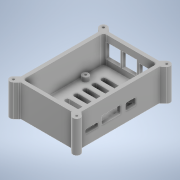
# Autodesk Inventor part: Case RevB Short
Saved by Autodesk Inventor 2021 (Build 250183000, 183)
## iProperties
Created: 2021-07-24
Part Number: Case RevB Short
Material: ABS Plastic
Document SubType Name: Modeling
Designer: cmzgt
Density: 0.1 g/cm^3
Appearance: Smooth - White
Author: cmzgt
## iProperties of the stored document _3DPrint.ipt
Created: 2021-07-24
Part Number: _3DPrint
Material: Generic
Document SubType Name: Modeling
Designer: cmzgt
Density: 1 g/cm^3
Appearance: Default
Author: cmzgt
Autodesk Inventor part; units mm, degrees
ref_plane "YZ Plane" through (0, 0, 0) normal (1, 0, 0) x (0, 1, 0)
ref_plane "XZ Plane" through (0, 0, 0) normal (0, 1, 0) x (-1, 0, 0)
ref_plane "XY Plane" through (0, 0, 0) normal (0, 0, 1) x (1, 0, 0)
sketch "Sketch1" plane through (0, 0, 0) normal (0, 1, 0) x (-1, 0, 0)
  line L0 (-33.3, -48.25) -> (33.3, -48.25)
  line L1 (33.3, -48.25) -> (33.3, 48.25)
  line L2 (33.3, 48.25) -> (-33.3, 48.25)
  line L3 (-33.3, 48.25) -> (-33.3, -48.25)
  line L4 (-33.3, -48.25) -> (33.3, 48.25) construction
  line L5 (33.3, -48.25) -> (-33.3, 48.25) construction
  point P0 (0, 0)
  dimension "d0" = 66.6
  dimension "d1" = 96.5
  constraints: 12 end point, 2 midpoint, 2 parallel, 1 horizontal, 1 perpendicular
  measures "d0" distance of L2.end L1.end
  measures "d1" distance of L0.end L1.end
extrude "Extrusion1" add sketch "Sketch1" along normal blind 5.08
sketch "Sketch2" plane through (0, 5.08, 0) normal (0, 1, 0) x (1, 0, 0)
  line L0 (29.5, 44.45) -> (-29.5, 44.45)
  line L1 (-29.5, 44.45) -> (-29.5, -44.45)
  line L2 (-29.5, -44.45) -> (29.5, -44.45)
  line L3 (29.5, -44.45) -> (29.5, 44.45)
  line L4 (29.5, 44.45) -> (-29.5, -44.45) construction
  line L5 (-29.5, 44.45) -> (29.5, -44.45) construction
  line L6 (-33.3, 48.25) -> (-33.3, -48.25) projected
  line L7 (-33.3, -48.25) -> (33.3, -48.25) projected
  line L8 (33.3, 48.25) -> (-33.3, 48.25) projected
  line L9 (33.3, -48.25) -> (33.3, 48.25) projected
  line L10 (25.7, -40.65) -> (33.3, -48.25) construction
  line L11 (23.8431, -44.45) -> (30.4716, -51.0784)
  line L12 (36.1284, -45.4216) -> (29.5, -38.7931)
  arc A0 (30.4716, -51.0784) -> (36.1284, -45.4216) centre (33.3, -48.25) ccw
  circle A1 centre (33.3, -48.25) radius 1.375
  point P0 (0, 0)
  dimension "d4" = 3.8
  dimension "d5" = 3.8
  dimension "d22" = 8
  dimension "d23" = 2.75
  constraints: 20 end point, 4 parallel, 3 midpoint, 2 centre point, 2 point on circle, 2 point on line, 2 tangent, 1 coincident, 1 horizontal, 1 perpendicular
  measures "d4" distance between parallel lines of L6 L1
  measures "d5" distance between parallel lines of L7 L2
  measures "d22" diameter of A0
  measures "d23" diameter of A1
extrude "Extrusion2" add sketch "Sketch2" along normal blind 30 contours L0 L1 L2 L11 L7 L6 L8 L9 L12 L3 | L12 L9 A1 L7 L11 L2 L3 | L9 L7 A1 picked at (32.8154, -47.4787)
sketch "Sketch3" plane through (0, 5.08, 0) normal (0, 1, 0) x (1, 0, 0)
  line L0 (29.5, -44.45) -> (-29.5, -44.45) construction
  line L1 (0, -44.45) -> (0, 44.45) construction
  line L2 (29.5, 44.45) -> (-29.5, 44.45) construction
  circle A0 centre (-24.5, -38.45) radius 3.5
  circle A1 centre (-24.5, -38.45) radius 1.375
  line L3 (29.5, 44.45) -> (29.5, -44.45) construction
  line L4 (29.5, 0) -> (-29.5, 0) construction
  line L5 (-29.5, -44.45) -> (-29.5, 44.45) construction
  circle A2 centre (-24.5, 19.55) radius 3.5
  circle A3 centre (-24.5, 19.55) radius 1.375
  circle A4 centre (24.5, -38.45) radius 3.5
  circle A5 centre (24.5, -38.45) radius 1.375
  circle A6 centre (24.5, 19.55) radius 3.5
  circle A7 centre (24.5, 19.55) radius 1.375
  point P0 (0, 0)
  dimension "d8" = 7
  dimension "d9" = 2.75
  dimension "d10" = 6
  dimension "d11" = 24.5
  dimension "d14" = 58
  constraints: 8 centre point, 4 coincident, 4 end point, 4 midpoint, 4 symmetric about line, 1 vertical, 8 other
  measures "d8" diameter of A0
  measures "d9" diameter of A1
  measures "d10" distance from line of L0 A0.centre
  measures "d11" distance from line of L1 A1.centre
  measures "d14" distance of A0.centre A2.centre
extrude "Extrusion3" add sketch "Sketch3" along normal blind 5
sketch "Sketch4" plane through (0, 0, 0) normal (0, -1, 0) x (1, 0, 0)
  line L0 (31.7938, 46.9342) -> (34.8062, 49.5658) construction
  line L1 (33.3, 48.25) -> (33.3, -48.25) projected
  line L2 (33.3, 42.9386) -> (37.4378, 46.5534)
  line L3 (32.1745, 52.5782) -> (29.1622, 49.9466)
  arc A0 (29.1622, 49.9466) -> (28.0164, 48.25) centre (31.7938, 46.9342) ccw
  arc A1 (37.4378, 46.5534) -> (32.1745, 52.5782) centre (34.8062, 49.5658) ccw
  line L4 (-33.3, 48.25) -> (33.3, 48.25) projected
  line L5 (28.0164, 48.25) -> (33.3, 48.25)
  line L6 (33.3, 48.25) -> (33.3, 42.9386)
  circle A2 centre (34.8062, 49.5658) radius 1.375
  line L7 (0, 48.25) -> (0, -48.25) construction
  line L8 (33.3, -48.25) -> (-33.3, -48.25) construction
  line L9 (33.3, 0) -> (-33.3, 0) construction
  line L10 (33.3, -48.25) -> (33.3, 48.25)
  line L11 (33.3, -42.9386) -> (37.4378, -46.5534)
  line L12 (32.1745, -52.5782) -> (29.1622, -49.9466)
  arc A3 (28.0164, -48.25) -> (29.1622, -49.9466) centre (31.7938, -46.9342) ccw
  arc A4 (32.1745, -52.5782) -> (37.4378, -46.5534) centre (34.8062, -49.5658) ccw
  line L13 (-33.3, -48.25) -> (33.3, -48.25)
  circle A5 centre (34.8062, -49.5658) radius 1.375
  line L14 (-33.3, 48.25) -> (-33.3, -48.25)
  line L15 (-33.3, 42.9386) -> (-37.4378, 46.5534)
  line L16 (-32.1745, 52.5782) -> (-29.1622, 49.9466)
  arc A6 (-28.0164, 48.25) -> (-29.1622, 49.9466) centre (-31.7938, 46.9342) ccw
  arc A7 (-32.1745, 52.5782) -> (-37.4378, 46.5534) centre (-34.8062, 49.5658) ccw
  line L17 (-28.0164, 48.25) -> (-33.3, 48.25)
  circle A8 centre (-34.8062, 49.5658) radius 1.375
  arc A9 (-37.4378, -46.5534) -> (-32.1745, -52.5782) centre (-34.8062, -49.5658) ccw
  line L18 (-33.3, -42.9386) -> (-37.4378, -46.5534)
  line L19 (-32.1745, -52.5782) -> (-29.1622, -49.9466)
  arc A10 (-29.1622, -49.9466) -> (-28.0164, -48.25) centre (-31.7938, -46.9342) ccw
  circle A11 centre (-34.8062, -49.5658) radius 1.375
  line L20 (-28.0164, -48.25) -> (-33.3, -48.25)
  line L21 (-33.3, -48.25) -> (-33.3, 48.25)
  point P0 (0, 0)
  point P1 (-28.0164, -48.25)
  point P2 (-33.3, -42.9386)
  point P3 (-28.0164, 48.25)
  point P4 (33.3, -42.9386)
  dimension "d24" = 2
  dimension "d25" = 8
  dimension "d26" = 131.141
  dimension "d27" = 2.75
  constraints: 40 end point, 30 symmetric about line, 16 point on circle, 12 centre point, 6 point on line, 4 coincident, 4 midpoint, 4 tangent, 1 collinear, 1 horizontal, 1 parallel, 9 other
  measures "d24" distance of L1.start L0.end
  measures "d25" diameter of A1
  measures "d26" angle of L1 L2
  measures "d27" diameter of A2
extrude "Extrusion4" add sketch "Sketch4" against normal up to surface (35.08 mm away) contours L4 A0 L3 A1 L2 L1 | L11 A4 L12 A3 L13 L1 | L4 L14 L15 A7 L16 A6 | A10 L19 A9 L18 L14 L13
fillet "Fillet2" radius 3 4 edges at (29.5, 20.08, -44.45) (-29.5, 20.08, -44.45) (-29.5, 20.08, 44.45) (29.5, 20.08, 44.45)
sketch "Sketch5" plane through (0, 5.08, 0) normal (0, 1, 0) x (1, 0, 0)
  line L0 (15, 0) -> (-15, 0) construction
  line L1 (15, 2.5) -> (-15, 2.5)
  line L2 (-15, -2.5) -> (15, -2.5)
  arc A0 (15, -2.5) -> (15, 2.5) centre (15, 0) ccw
  arc A1 (-15, 2.5) -> (-15, -2.5) centre (-15, 0) ccw
  line L3 (-26.5, -44.45) -> (26.5, -44.45) construction
  line L4 (0, -44.45) -> (0, 44.45) construction
  line L5 (-26.5, 44.45) -> (26.5, 44.45) construction
  arc A2 (-15, 12.5) -> (-15, 7.5) centre (-15, 10) ccw
  line L6 (15, 12.5) -> (-15, 12.5)
  line L7 (-15, 7.5) -> (15, 7.5)
  arc A3 (15, 7.5) -> (15, 12.5) centre (15, 10) ccw
  arc A4 (-15, 22.5) -> (-15, 17.5) centre (-15, 20) ccw
  line L8 (15, 22.5) -> (-15, 22.5)
  line L9 (-15, 17.5) -> (15, 17.5)
  arc A5 (15, 17.5) -> (15, 22.5) centre (15, 20) ccw
  arc A6 (-15, 32.5) -> (-15, 27.5) centre (-15, 30) ccw
  line L10 (15, 32.5) -> (-15, 32.5)
  line L11 (-15, 27.5) -> (15, 27.5)
  arc A7 (15, 27.5) -> (15, 32.5) centre (15, 30) ccw
  arc A8 (-15, -7.5) -> (-15, -12.5) centre (-15, -10) ccw
  line L12 (-15, -12.5) -> (15, -12.5)
  line L13 (15, -7.5) -> (-15, -7.5)
  arc A9 (15, -12.5) -> (15, -7.5) centre (15, -10) ccw
  arc A10 (-15, -17.5) -> (-15, -22.5) centre (-15, -20) ccw
  line L14 (-15, -22.5) -> (15, -22.5)
  line L15 (15, -17.5) -> (-15, -17.5)
  arc A11 (15, -22.5) -> (15, -17.5) centre (15, -20) ccw
  arc A12 (-15, -27.5) -> (-15, -32.5) centre (-15, -30) ccw
  line L16 (-15, -32.5) -> (15, -32.5)
  line L17 (15, -27.5) -> (-15, -27.5)
  arc A13 (15, -32.5) -> (15, -27.5) centre (15, -30) ccw
  point P0 (0, 0)
  dimension "d31" = 15
  dimension "d32" = 5
  dimension "d35" = 10
  dimension "d42" = 10
  constraints: 34 end point, 28 point on circle, 14 centre point, 4 tangent, 3 midpoint, 2 vertical, 1 horizontal, 1 parallel, 60 other
  measures "d31" distance of point (0, 0) L0.end
  measures "d32" diameter of A1
  measures "d35" distance of L0.end A2.centre
  measures "d42" distance of L0.end A8.centre
extrude "Extrusion5" cut sketch "Sketch5" against normal up to surface (5.08 mm away)
sketch "Sketch9" plane through (28.0164, 0, -48.25) normal (0, 0, -1) x (-1, 0, 0)
  line L0 (7.0164, 10.08) -> (0.0164, 10.08) projected
  line L1 (2.1414, 10.08) -> (4.8914, 10.08) projected
  line L2 (2.1414, 10.08) -> (4.8914, 10.08) construction
  line L3 (3.5164, 10.08) -> (0.0164, 10.08) construction
  line L4 (7.0164, 10.08) -> (0.0164, 10.08) projected
  line L5 (0, 35.08) -> (0, 0) projected
  line L6 (0.0164, 10.08) -> (0, 13.58) construction
  line L7 (18.375, 11.35) -> (2.125, 11.35)
  line L8 (2.125, 11.35) -> (2.125, 25.6)
  line L9 (2.125, 25.6) -> (18.375, 25.6)
  line L10 (18.375, 25.6) -> (18.375, 11.35)
  line L11 (10.25, 25.6) -> (10.25, 11.35) construction
  line L12 (21, 11.35) -> (37, 11.35)
  line L13 (37, 11.35) -> (37, 27.85)
  line L14 (37, 27.85) -> (21, 27.85)
  line L15 (21, 27.85) -> (21, 11.35)
  line L16 (29, 27.85) -> (29, 11.35) construction
  line L17 (55, 27.85) -> (39, 27.85)
  line L18 (55, 11.35) -> (55, 27.85)
  line L19 (39, 11.35) -> (55, 11.35)
  line L20 (39, 27.85) -> (39, 11.35)
  point P0 (28.0164, 0)
  point P1 (47, 27.85)
  point P2 (47, 11.35)
  dimension "d58" = 3.5
  dimension "d60" = 3.5
  dimension "d63" = 16.25
  dimension "d64" = 14.25
  dimension "d65" = 1.27
  dimension "d66" = 10.25
  dimension "d69" = 16
  dimension "d70" = 16.5
  dimension "d71" = 1.27
  dimension "d72" = 29
  dimension "d75" = 18
  constraints: 32 end point, 5 midpoint, 4 parallel, 3 horizontal, 2 perpendicular, 1 collinear, 1 point on line, 10 other
  measures "d58" distance of L3.start L0.end
  measures "d60" distance of L0.end L6.end
  measures "d63" distance of L8.end L9.end
  measures "d64" distance of L7.end L8.end
  measures "d65" distance between parallel lines of L0 L7
  measures "d66" distance between parallel lines of L5 L11
  measures "d69" distance of L14.end L13.end
  measures "d70" distance of L12.end L13.end
  measures "d71" distance between parallel lines of L4 L12
  measures "d72" distance between parallel lines of L5 L16
  measures "d75" distance of L13.end L17.start
extrude "Extrusion7" cut sketch "Sketch9" against normal up to surface (3.8 mm away)
sketch "Sketch11" plane through (33.3, 0, 42.9386) normal (1, 0, 0) x (0, 0, -1)
  line L0 (4.5402, 15.78) -> (18.5209, 15.78)
  line L1 (18.5209, 15.78) -> (18.5209, 10.78)
  line L2 (18.5209, 10.78) -> (4.5402, 10.78)
  line L3 (4.5402, 10.78) -> (4.5402, 15.78)
  line L4 (22.4305, 19.78) -> (43.4305, 19.78)
  line L5 (43.4305, 19.78) -> (43.4305, 10.78)
  line L6 (43.4305, 10.78) -> (22.4305, 10.78)
  line L7 (22.4305, 10.78) -> (22.4305, 19.78)
  line L8 (25.4305, 16.69) -> (25.4305, 14.2116)
  line L9 (40.4305, 14.2116) -> (40.4305, 16.69)
  line L10 (15.5209, 13.09) -> (15.5209, 12.8971)
  line L11 (7.5402, 12.8971) -> (7.5402, 13.09)
  line L12 (82.9128, 10.28) -> (3.9886, 10.28)
  line L13 (49.0305, 18.78) -> (60.0305, 18.78)
  line L14 (60.0305, 18.78) -> (60.0305, 10.78)
  line L15 (60.0305, 10.78) -> (49.0305, 10.78)
  line L16 (49.0305, 10.78) -> (49.0305, 18.78)
  line L17 (51.0305, 17.41) -> (51.0305, 11.41)
  line L18 (58.0305, 11.41) -> (58.0305, 17.41)
  point P0 (42.9386, 0)
extrude "Extrusion8" cut sketch "Sketch11" against normal up to surface (3.8 mm away)
fillet "Fillet4" radius 1 12 edges at (31.4, 19.78, -0.492) (31.4, 19.78, 20.508) (31.4, 10.78, 20.508) (31.4, 10.78, -0.492) (31.4, 18.78, -6.092) (31.4, 10.78, -6.092) (31.4, 10.78, -17.092) (31.4, 18.78, -17.092) (31.4, 15.78, 24.4177) (31.4, 15.78, 38.3984) (31.4, 10.78, 38.3984) (31.4, 10.78, 24.4177)
body "Solid1"
